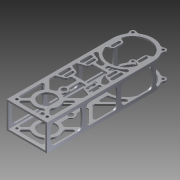
# Autodesk Inventor part: upper gearbox frame 5
Saved by Autodesk Inventor 2012 (Build 160160000, 160)
## iProperties
Created: 2013-09-11
Part Number: upper gearbox frame 5
Material: Default
Document SubType Name: Modeling
Designer: Bryce
Density: 1 g/cm^3
Author: Bryce
Autodesk Inventor part; units mm, degrees
ref_plane "YZ Plane" through (0, 0, 0) normal (1, 0, 0) x (0, 1, 0)
ref_plane "XZ Plane" through (0, 0, 0) normal (0, 1, 0) x (-1, 0, 0)
ref_plane "XY Plane" through (0, 0, 0) normal (0, 0, 1) x (1, 0, 0)
sketch "Sketch1" plane through (0, 0, 0) normal (0, 0, 1) x (1, 0, 0)
  line L0 (0, 0) -> (76.2, 0)
  line L1 (76.2, 0) -> (76.2, 50.8)
  line L2 (76.2, 50.8) -> (0, 50.8)
  line L3 (0, 50.8) -> (0, 0)
  line L4 (3.175, 3.175) -> (73.025, 3.175)
  line L5 (73.025, 3.175) -> (73.025, 47.625)
  line L6 (73.025, 47.625) -> (3.175, 47.625)
  line L7 (3.175, 47.625) -> (3.175, 3.175)
  dimension "d0" = 50.8
  dimension "d1" = 76.2
  dimension "d2" = 3.175
  dimension "d3" = 3.175
  dimension "d4" = 3.175
  dimension "d5" = 3.175
  constraints: 16 end point, 4 parallel, 2 horizontal, 2 perpendicular
  measures "d0" distance of L2.end L0.start
  measures "d1" distance of L0.start L0.end
  measures "d2" distance between parallel lines of L0 L4
  measures "d3" distance between parallel lines of L3 L7
  measures "d4" distance between parallel lines of L2 L6
  measures "d5" distance between parallel lines of L1 L5
extrude "Extrusion1" add sketch "Sketch1" along normal blind 254
sketch "Sketch2" plane through (0, 0, 0) normal (0, -1, 0) x (1, 0, 0)
  line L0 (76.2, 254) -> (0, 254) projected
  line L1 (0, 0) -> (0, 254) projected
  line L2 (0, 0) -> (76.2, 0) projected
  line L3 (76.2, 0) -> (76.2, 254) projected
  circle A0 centre (38.1, 215.9) radius 15.875
  arc A1 (71.4375, 66.675) -> (4.7625, 66.675) centre (38.1, 66.675) ccw
  arc A2 (4.7625, 53.975) -> (71.4375, 53.975) centre (38.1, 53.975) ccw
  circle A3 centre (38.1, 171.45) radius 4.6482
  line L4 (38.1, 215.9) -> (0, 254) construction
  line L5 (38.1, 215.9) -> (76.2, 254) construction
  line L6 (38.1, 215.9) -> (0, 177.8) construction
  line L7 (38.1, 215.9) -> (76.2, 177.8) construction
  arc A4 (20.3007, 229.2092) -> (20.3007, 202.5908) centre (38.1, 215.9) ccw
  arc A5 (51.4092, 233.6993) -> (24.7908, 233.6993) centre (38.1, 215.9) ccw
  arc A6 (55.8993, 202.5908) -> (55.8993, 229.2092) centre (38.1, 215.9) ccw
  arc A7 (24.7908, 198.1007) -> (34.925, 193.903) centre (38.1, 215.9) ccw
  line L8 (6.35, 243.1599) -> (6.35, 188.6401)
  line L9 (10.8401, 247.65) -> (65.3599, 247.65)
  line L10 (69.85, 243.1599) -> (69.85, 188.6401)
  line L11 (6.35, 243.1599) -> (20.3007, 229.2092)
  line L12 (20.3007, 202.5908) -> (6.35, 188.6401)
  line L13 (24.7908, 233.6993) -> (10.8401, 247.65)
  line L14 (51.4092, 233.6993) -> (65.3599, 247.65)
  line L15 (69.85, 243.1599) -> (55.8993, 229.2092)
  line L16 (55.8993, 202.5908) -> (69.85, 188.6401)
  line L17 (6.35, 179.6599) -> (6.35, 168.4676)
  line L18 (69.85, 179.6599) -> (69.85, 168.4676)
  arc A8 (69.85, 87.7356) -> (41.275, 104.6425) centre (38.1, 66.675) ccw
  line L19 (6.35, 179.6599) -> (24.7908, 198.1007)
  line L20 (51.4092, 198.1007) -> (69.85, 179.6599)
  arc A9 (34.925, 178.7248) -> (34.925, 164.1752) centre (38.1, 171.45) ccw
  arc A10 (41.275, 164.1752) -> (41.275, 178.7248) centre (38.1, 171.45) ccw
  line L21 (38.1, 215.9) -> (38.1, 171.45) construction
  line L22 (38.1, 171.45) -> (38.1, 66.675) construction
  line L23 (34.925, 178.7248) -> (34.925, 193.903)
  line L24 (41.275, 193.903) -> (41.275, 178.7248)
  line L25 (34.925, 164.1752) -> (34.925, 139.8926)
  line L26 (41.275, 164.1752) -> (41.275, 139.8926)
  arc A11 (41.275, 193.903) -> (51.4092, 198.1007) centre (38.1, 215.9) ccw
  arc A12 (34.925, 193.903) -> (41.275, 193.903) centre (38.1, 215.9) ccw
  arc A13 (41.275, 104.6425) -> (34.925, 104.6425) centre (38.1, 66.675) ccw construction
  arc A14 (34.925, 104.6425) -> (6.35, 87.7356) centre (38.1, 66.675) ccw
  line L27 (4.7625, 66.675) -> (4.7625, 53.975)
  line L28 (71.4375, 66.675) -> (71.4375, 53.975)
  arc A15 (0, 53.975) -> (5.274, 34.6342) centre (38.1, 53.975) ccw
  line L29 (76.2, 95.25) -> (38.1, 133.35) construction
  line L30 (0, 95.25) -> (38.1, 133.35) construction
  line L31 (38.1, 133.35) -> (0, 171.45) construction
  line L32 (38.1, 133.35) -> (76.2, 171.45) construction
  line L33 (41.4676, 133.35) -> (69.85, 161.7324)
  line L34 (41.4676, 133.35) -> (69.85, 104.9676)
  line L35 (69.85, 98.2324) -> (41.275, 126.8074)
  line L36 (38.1, 129.9824) -> (34.925, 126.8074) construction
  line L37 (6.35, 104.9676) -> (34.7324, 133.35)
  line L38 (34.7324, 133.35) -> (6.35, 161.7324)
  line L39 (6.35, 168.4676) -> (34.925, 139.8926)
  line L40 (38.1, 136.7176) -> (41.275, 139.8926)
  line L41 (41.275, 139.8926) -> (41.275, 126.8074) construction
  line L42 (41.275, 126.8074) -> (41.275, 104.6425)
  line L43 (34.925, 126.8074) -> (34.925, 104.6425)
  line L44 (34.925, 139.8926) -> (34.925, 126.8074) construction
  line L45 (34.925, 126.8074) -> (6.35, 98.2324)
  line L46 (41.275, 126.8074) -> (38.1, 129.9824) construction
  line L47 (41.275, 139.8926) -> (69.85, 168.4676)
  line L48 (34.925, 139.8926) -> (38.1, 136.7176)
  line L49 (69.85, 161.7324) -> (69.85, 104.9676)
  line L50 (69.85, 168.4676) -> (69.85, 161.7324) construction
  line L51 (6.35, 168.4676) -> (6.35, 161.7324) construction
  line L52 (6.35, 161.7324) -> (6.35, 104.9676)
  line L53 (6.35, 104.9676) -> (6.35, 98.2324) construction
  line L54 (6.35, 98.2324) -> (6.35, 87.7356)
  line L55 (69.85, 98.2324) -> (69.85, 87.7356)
  line L56 (69.85, 104.9676) -> (69.85, 98.2324) construction
  circle A16 centre (66.675, 244.475) radius 2.5527
  circle A17 centre (66.675, 25.4) radius 2.5527
  arc A18 (64.0036, 21.0791) -> (57.4408, 21.149) centre (60.6643, 15.6781) ccw
  arc A19 (70.926, 34.6342) -> (70.9959, 28.0714) centre (76.3969, 31.4107) ccw
  arc A20 (64.0036, 21.0791) -> (70.9959, 28.0714) centre (66.675, 25.4) ccw
  arc A21 (70.926, 34.6342) -> (76.2, 53.975) centre (38.1, 53.975) ccw
  circle A22 centre (9.525, 25.4) radius 2.5527
  arc A23 (5.2041, 28.0714) -> (12.1964, 21.0791) centre (9.525, 25.4) ccw
  arc A24 (5.2041, 28.0714) -> (5.274, 34.6342) centre (-0.1969, 31.4107) ccw
  arc A25 (18.7592, 21.149) -> (12.1964, 21.0791) centre (15.5357, 15.6781) ccw
  arc A26 (18.7592, 21.149) -> (57.4408, 21.149) centre (38.1, 53.975) ccw
  circle A27 centre (9.525, 244.475) radius 2.5527
  dimension "d62" = 12.7
  dimension "d8" = 31.75
  dimension "d9" = 38.1
  dimension "d10" = 38.1
  dimension "d11" = 33.3375
  dimension "d15" = 38.1
  dimension "d18" = 12.7
  dimension "d30" = 9.2964
  dimension "d31" = 44.45
  dimension "d32" = 3.175
  dimension "d33" = 3.175
  dimension "d34" = 3.175
  dimension "d35" = 3.175
  dimension "d36" = 3.175
  dimension "d37" = 3.175
  dimension "d38" = 6.35
  dimension "d39" = 6.35
  dimension "d41" = 6.35
  dimension "d42" = 22.225
  dimension "d43" = 38.1
  dimension "d44" = 3.175
  dimension "d45" = 3.175
  dimension "d46" = 3.175
  dimension "d47" = 3.175
  dimension "d48" = 7.9375
  dimension "d202" = 120.65
  dimension "d203" = 45
  dimension "d204" = 2.3813
  dimension "d205" = 4.7625
  dimension "d206" = 4.7625
  dimension "d211" = 9.525
  dimension "d212" = 5.1054
  dimension "d213" = 228.6
  dimension "d214" = 9.525
  dimension "d216" = 6.35
  dimension "d218" = 9.525
  dimension "d237" = 187.325
  dimension "d238" = 5.08
  constraints: 106 end point, 63 parallel, 48 point on circle, 28 centre point, 25 collinear, 21 point on line, 16 perpendicular, 14 tangent, 11 equal radius, 10 coincident, 2 horizontal alignment, 1 vertical alignment
  measures "d8" diameter of A0
  measures "d9" distance from line of L1 L4.start
  measures "d10" distance from line of L0 L4.start
  measures "d11" radius of A1
  measures "d15" distance from line of L1 A1.centre
  measures "d18" distance of A1.centre A2.centre
  measures "d30" diameter of A3
  measures "d31" distance of L4.start A3.centre
  measures "d32" distance between parallel lines of L4 L11
  measures "d33" distance between parallel lines of L12 L6
  measures "d34" distance between parallel lines of L5 L14
  measures "d35" distance between parallel lines of L15 L5
  measures "d36" distance between parallel lines of L7 L16
  measures "d37" distance between parallel lines of L4 L13
  measures "d38" distance between parallel lines of L1 L8
  measures "d39" distance between parallel lines of L0 L9
  measures "d41" distance between parallel lines of L3 L10
  measures "d42" radius of A6
  measures "d43" radius of A8
  measures "d44" distance between parallel lines of L6 L19
  measures "d45" distance between parallel lines of L7 L20
  measures "d46" distance between parallel lines of L22 L25
  measures "d47" distance between parallel lines of L26 L22
  measures "d48" radius of A10
  measures "d202" distance from line of L0 L29.end
  measures "d203" angle of L3 L29
  measures "d204" distance between parallel lines of L29 L34
  measures "d205" distance between parallel lines of L34 L35
  measures "d206" distance between parallel lines of L37 L36
  measures "d211" distance from line of L0 A16.centre
  measures "d212" diameter of A16
  measures "d213" distance from line of L0 A17.centre
  measures "d214" distance from line of L3 A17.centre
  measures "d216" radius of A19
  measures "d218" distance from line of L1 A22.centre
  measures "d237" distance from line of L0 L22.end
  measures "d238" radius of A20
extrude "Extrusion2" cut sketch "Sketch2" against normal blind 6.35 contours A0 | L28 A2 L27 A1 | A3 | A4 L12 L8 L11 | A5 L13 L9 L14 | A6 L15 L10 L16 | A7 L23 A9 L25 L39 L17 L19 | A11 L20 L18 L47 L26 A10 L24 | A8 L42 L35 L55 | A14 L54 L45 L43 | L33 L49 L34 | L52 L38 L37
fillet "Fillet1" radius 3.175 40 edges at (6.35, 1.5875, 87.7356) (69.85, 1.5875, 87.7356) (34.925, 1.5875, 104.6425) (41.275, 1.5875, 104.6425) (6.35, 1.5875, 243.1599) (6.35, 1.5875, 188.6401) (6.35, 1.5875, 179.6599) (10.8401, 1.5875, 247.65) (20.3007, 1.5875, 229.2092) (20.3007, 1.5875, 202.5908) (24.7908, 1.5875, 233.6993) (34.925, 1.5875, 193.903) (34.925, 1.5875, 178.7248) (34.925, 1.5875, 164.1752) (41.275, 1.5875, 193.903) (41.275, 1.5875, 178.7248) (41.275, 1.5875, 164.1752) (51.4092, 1.5875, 233.6993) (55.8993, 1.5875, 229.2092) (51.4092, 1.5875, 198.1007) (55.8993, 1.5875, 202.5908) (65.3599, 1.5875, 247.65) (69.85, 1.5875, 243.1599) (69.85, 1.5875, 188.6401) (69.85, 1.5875, 179.6599) (24.7908, 1.5875, 198.1007) (69.85, 1.5875, 168.4676) (6.35, 1.5875, 168.4676) (69.85, 1.5875, 161.7324) (6.35, 1.5875, 161.7324) (41.275, 1.5875, 139.8926) (34.925, 1.5875, 139.8926) (41.4676, 1.5875, 133.35) (34.7324, 1.5875, 133.35) (41.275, 1.5875, 126.8074) (34.925, 1.5875, 126.8074) (69.85, 1.5875, 104.9676) (6.35, 1.5875, 104.9676) (69.85, 1.5875, 98.2324) (6.35, 1.5875, 98.2324)
sketch "Sketch3" plane through (0, 50.8, 0) normal (0, 1, 0) x (1, 0, 0)
  line L0 (0, -254) -> (76.2, -254) projected
  line L1 (76.2, 0) -> (76.2, -254) projected
  line L2 (76.2, 0) -> (0, 0) projected
  line L3 (0, 0) -> (0, -254) projected
  circle A0 centre (38.1, -215.9) radius 15.875 projected
  arc A1 (20.32, -106.68) -> (15.24, -106.68) centre (17.78, -106.68) ccw
  arc A2 (15.24, -119.38) -> (20.32, -119.38) centre (17.78, -119.38) ccw
  line L4 (20.32, -106.68) -> (20.32, -119.38)
  line L5 (15.24, -106.68) -> (15.24, -119.38)
  arc A3 (60.96, -106.68) -> (55.88, -106.68) centre (58.42, -106.68) ccw
  arc A4 (55.88, -119.38) -> (60.96, -119.38) centre (58.42, -119.38) ccw
  line L6 (60.96, -106.68) -> (60.96, -119.38)
  line L7 (55.88, -106.68) -> (55.88, -119.38)
  arc A5 (20.32, -147.32) -> (15.24, -147.32) centre (17.78, -147.32) ccw
  arc A6 (15.24, -160.02) -> (20.32, -160.02) centre (17.78, -160.02) ccw
  line L8 (20.32, -147.32) -> (20.32, -160.02)
  line L9 (15.24, -147.32) -> (15.24, -160.02)
  arc A7 (60.96, -147.32) -> (55.88, -147.32) centre (58.42, -147.32) ccw
  line L10 (60.96, -147.32) -> (60.96, -160.02)
  line L11 (55.88, -147.32) -> (55.88, -160.02)
  arc A8 (55.88, -160.02) -> (60.96, -160.02) centre (58.42, -160.02) ccw
  arc A9 (50.8, -127) -> (25.4, -127) centre (38.1, -127) ccw construction
  line L12 (50.8, -127) -> (50.8, -139.7) construction
  line L13 (25.4, -127) -> (25.4, -139.7) construction
  arc A10 (25.4, -139.7) -> (50.8, -139.7) centre (38.1, -139.7) ccw construction
  arc A11 (15.24, -53.975) -> (10.16, -53.975) centre (12.7, -53.975) ccw
  arc A12 (66.04, -53.975) -> (60.96, -53.975) centre (63.5, -53.975) ccw
  arc A13 (60.96, -66.675) -> (66.04, -66.675) centre (63.5, -66.675) ccw
  line L14 (10.16, -53.975) -> (10.16, -66.675)
  line L15 (15.24, -53.975) -> (15.24, -66.675)
  line L16 (60.96, -53.975) -> (60.96, -66.675)
  line L17 (66.04, -53.975) -> (66.04, -66.675)
  line L18 (12.7, -165.1) -> (63.5, -165.1) construction
  line L19 (63.5, -165.1) -> (63.5, -163.8962) construction
  line L20 (63.5, -101.6) -> (12.7, -101.6) construction
  line L21 (12.7, -101.6) -> (12.7, -102.8038) construction
  arc A14 (6.35, -87.7356) -> (69.85, -87.7356) centre (38.1, -66.675) ccw construction
  line L22 (6.35, -6.35) -> (69.85, -6.35) construction
  line L23 (69.85, -6.35) -> (69.85, -84.7055) construction
  line L24 (69.85, -247.65) -> (65.3599, -247.65) construction
  line L25 (6.35, -247.65) -> (6.35, -243.1599) construction
  arc A15 (10.16, -66.675) -> (15.24, -66.675) centre (12.7, -66.675) ccw
  arc A16 (76.2, -53.975) -> (0, -53.975) centre (38.1, -53.975) ccw
  circle A17 centre (38.1, -215.9) radius 31.75 construction
  circle A18 centre (38.1, -184.15) radius 4.6482
  arc A19 (24.7908, -233.6993) -> (51.4092, -233.6993) centre (38.1, -215.9) ccw
  line L26 (38.1, -215.9) -> (0, -254) construction
  line L27 (38.1, -215.9) -> (0, -177.8) construction
  line L28 (38.1, -215.9) -> (76.2, -254) construction
  line L29 (38.1, -215.9) -> (76.2, -177.8) construction
  line L30 (24.7908, -233.6993) -> (10.8401, -247.65)
  line L31 (51.4092, -233.6993) -> (65.3599, -247.65)
  line L32 (65.3599, -247.65) -> (10.8401, -247.65)
  line L33 (10.8401, -247.65) -> (6.35, -247.65) construction
  line L34 (20.3007, -229.2092) -> (6.35, -243.1599)
  line L35 (20.3007, -202.5908) -> (6.35, -188.6401)
  line L36 (24.7908, -198.1007) -> (6.35, -179.6599)
  line L37 (51.4092, -198.1007) -> (69.85, -179.6599)
  line L38 (55.8993, -202.5908) -> (69.85, -188.6401)
  line L39 (55.8993, -229.2092) -> (69.85, -243.1599)
  arc A20 (20.3007, -202.5908) -> (20.3007, -229.2092) centre (38.1, -215.9) ccw
  arc A21 (51.4092, -198.1007) -> (44.851, -194.7251) centre (38.1, -215.9) ccw
  arc A22 (55.8993, -229.2092) -> (55.8993, -202.5908) centre (38.1, -215.9) ccw
  line L40 (69.85, -188.6401) -> (69.85, -243.1599)
  line L41 (69.85, -243.1599) -> (69.85, -247.65) construction
  line L42 (6.35, -243.1599) -> (6.35, -188.6401)
  line L43 (6.35, -188.6401) -> (6.35, -179.6599) construction
  arc A23 (19.5175, -164.7936) -> (22.86, -160.02) centre (17.78, -160.02) ccw
  arc A24 (22.86, -147.32) -> (19.5175, -142.5464) centre (17.78, -147.32) ccw
  arc A25 (19.5175, -124.1536) -> (22.86, -119.38) centre (17.78, -119.38) ccw
  arc A26 (22.86, -106.68) -> (19.5175, -101.9064) centre (17.78, -106.68) ccw
  arc A27 (56.6825, -101.9064) -> (53.34, -106.68) centre (58.42, -106.68) ccw
  arc A28 (53.34, -119.38) -> (56.6825, -124.1536) centre (58.42, -119.38) ccw
  arc A29 (56.6825, -142.5464) -> (53.34, -147.32) centre (58.42, -147.32) ccw
  arc A30 (53.34, -160.02) -> (56.6825, -164.7936) centre (58.42, -160.02) ccw
  line L44 (22.86, -147.32) -> (22.86, -151.2887)
  line L45 (22.86, -106.68) -> (22.86, -110.6487)
  line L46 (53.34, -106.68) -> (53.34, -110.6487)
  line L47 (53.34, -147.32) -> (53.34, -151.2887)
  line L48 (19.5175, -142.5464) -> (6.35, -137.7538)
  line L49 (19.5175, -124.1536) -> (6.35, -128.9462)
  line L50 (56.6825, -124.1536) -> (69.85, -128.9462)
  line L51 (56.6825, -142.5464) -> (69.85, -137.7538)
  line L52 (19.5175, -101.9064) -> (6.35, -97.1138)
  line L53 (56.6825, -101.9064) -> (69.85, -97.1138)
  line L54 (19.5175, -164.7936) -> (6.35, -169.5862)
  line L55 (56.6825, -164.7936) -> (69.85, -169.5862)
  line L56 (22.86, -153.67) -> (53.34, -153.67) construction
  line L57 (22.86, -113.03) -> (53.34, -113.03) construction
  line L58 (22.86, -115.4112) -> (53.34, -115.4112)
  line L59 (22.86, -110.6487) -> (35.7188, -110.6487)
  line L60 (22.86, -151.2887) -> (53.34, -151.2887)
  line L61 (22.86, -156.0512) -> (35.7188, -156.0512)
  arc A31 (35.7188, -176.9116) -> (32.6538, -189.4795) centre (38.1, -184.15) ccw
  arc A32 (43.5462, -189.4795) -> (40.4813, -176.9116) centre (38.1, -184.15) ccw
  line L62 (38.1, -153.67) -> (38.1, -184.15) construction
  line L63 (35.7188, -156.0512) -> (35.7188, -176.9116)
  line L64 (40.4813, -156.0512) -> (40.4813, -176.9116)
  arc A33 (31.349, -194.7251) -> (32.6538, -189.4795) centre (30.3846, -191.7002) ccw
  arc A34 (31.349, -194.7251) -> (24.7908, -198.1007) centre (38.1, -215.9) ccw
  arc A35 (44.851, -194.7251) -> (31.349, -194.7251) centre (38.1, -215.9) ccw construction
  line L65 (35.7188, -156.0512) -> (40.4813, -156.0512) construction
  line L66 (40.4813, -156.0512) -> (53.34, -156.0512)
  line L67 (6.35, -169.5862) -> (6.35, -141.1326)
  line L68 (6.35, -179.6599) -> (6.35, -169.5862)
  line L69 (69.85, -179.6599) -> (69.85, -188.6401) construction
  line L70 (69.85, -169.5862) -> (69.85, -179.6599)
  line L71 (69.85, -137.7538) -> (69.85, -141.1326) construction
  line L72 (6.35, -137.7538) -> (6.35, -128.9462)
  line L73 (69.85, -128.9462) -> (69.85, -137.7538)
  arc A36 (69.85, -53.975) -> (68.9758, -46.5759) centre (38.1, -53.975) ccw construction
  arc A37 (14.4375, -71.4486) -> (17.78, -66.675) centre (12.7, -66.675) ccw
  arc A38 (17.78, -53.975) -> (14.4375, -49.2014) centre (12.7, -53.975) ccw
  arc A39 (61.7625, -49.2014) -> (58.42, -53.975) centre (63.5, -53.975) ccw
  arc A40 (58.42, -66.675) -> (61.7625, -71.4486) centre (63.5, -66.675) ccw
  line L74 (17.78, -53.975) -> (17.78, -66.675)
  line L75 (58.42, -53.975) -> (58.42, -66.675)
  line L76 (14.4375, -71.4486) -> (7.2242, -74.0741)
  line L77 (14.4375, -49.2014) -> (7.2242, -46.5759)
  line L78 (61.7625, -49.2014) -> (68.9758, -46.5759)
  line L79 (61.7625, -71.4486) -> (68.9758, -74.0741)
  arc A41 (6.35, -66.675) -> (7.2242, -74.0741) centre (38.1, -66.675) ccw construction
  arc A42 (7.2242, -74.0741) -> (68.9758, -74.0741) centre (38.1, -66.675) ccw
  line L80 (7.2242, -74.0741) -> (10.16, -73.0055)
  arc A43 (68.9758, -74.0741) -> (69.85, -66.675) centre (38.1, -66.675) ccw construction
  arc A44 (7.2242, -46.5759) -> (6.35, -53.975) centre (38.1, -53.975) ccw construction
  arc A45 (68.9758, -46.5759) -> (7.2242, -46.5759) centre (38.1, -53.975) ccw
  arc A46 (6.35, -84.7055) -> (35.7188, -103.1098) centre (38.1, -66.675) ccw
  line L81 (38.1, -103.1875) -> (38.1, -110.6487) construction
  line L82 (35.7188, -103.1098) -> (35.7188, -110.6487)
  line L83 (40.4813, -110.6487) -> (40.4813, -103.1098)
  arc A47 (35.7188, -103.1098) -> (40.4813, -103.1098) centre (38.1, -66.675) ccw construction
  arc A48 (40.4813, -103.1098) -> (69.85, -84.7055) centre (38.1, -66.675) ccw
  line L84 (35.7188, -110.6487) -> (40.4813, -110.6487) construction
  line L85 (40.4813, -110.6487) -> (53.34, -110.6487)
  line L86 (22.86, -115.4112) -> (22.86, -119.38)
  line L87 (22.86, -110.6487) -> (22.86, -115.4112) construction
  line L88 (53.34, -110.6487) -> (53.34, -115.4112) construction
  line L89 (53.34, -115.4112) -> (53.34, -119.38)
  line L90 (22.86, -151.2887) -> (22.86, -156.0512) construction
  line L91 (22.86, -156.0512) -> (22.86, -160.02)
  line L92 (53.34, -156.0512) -> (53.34, -160.02)
  line L93 (53.34, -151.2887) -> (53.34, -156.0512) construction
  line L94 (6.35, -97.1138) -> (6.35, -84.7055)
  line L95 (6.35, -84.7055) -> (6.35, -6.35) construction
  line L96 (69.85, -84.7055) -> (69.85, -97.1138)
  line L97 (69.85, -97.1138) -> (69.85, -100.4926) construction
  line L98 (12.7, -163.8962) -> (6.35, -166.2074)
  line L99 (12.7, -143.4438) -> (6.35, -141.1326)
  line L100 (12.7, -123.2562) -> (6.35, -125.5674)
  line L101 (12.7, -102.8038) -> (6.35, -100.4926)
  line L102 (63.5, -102.8038) -> (69.85, -100.4926)
  line L103 (63.5, -123.2562) -> (69.85, -125.5674)
  line L104 (63.5, -163.8962) -> (69.85, -166.2074)
  line L105 (63.5, -143.4438) -> (69.85, -141.1326)
  line L106 (12.7, -163.8962) -> (12.7, -165.1) construction
  line L107 (12.7, -143.4438) -> (12.7, -163.8962)
  line L108 (63.5, -163.8962) -> (63.5, -143.4438)
  line L109 (63.5, -143.4438) -> (63.5, -123.2562) construction
  line L110 (12.7, -102.8038) -> (12.7, -123.2562)
  line L111 (12.7, -123.2562) -> (12.7, -143.4438) construction
  line L112 (63.5, -102.8038) -> (63.5, -101.6) construction
  line L113 (63.5, -123.2562) -> (63.5, -102.8038)
  line L114 (69.85, -100.4926) -> (69.85, -125.5674)
  line L115 (69.85, -125.5674) -> (69.85, -128.9462) construction
  line L116 (6.35, -100.4926) -> (6.35, -125.5674)
  line L117 (6.35, -100.4926) -> (6.35, -97.1138) construction
  line L118 (6.35, -125.5674) -> (6.35, -128.9462) construction
  line L119 (69.85, -141.1326) -> (69.85, -166.2074)
  line L120 (69.85, -166.2074) -> (69.85, -169.5862) construction
  line L121 (6.35, -141.1326) -> (6.35, -137.7538) construction
  circle A49 centre (38.1, -184.15) radius 15.875 construction
  arc A50 (43.5462, -189.4795) -> (44.851, -194.7251) centre (45.8154, -191.7002) ccw
  dimension "d91" = 63.5
  dimension "d52" = 12.7
  dimension "d53" = 2.54
  dimension "d54" = 12.7
  dimension "d55" = 2.54
  dimension "d56" = 12.7
  dimension "d57" = 2.54
  dimension "d58" = 12.7
  dimension "d59" = 2.54
  dimension "d60" = 40.64
  dimension "d61" = 40.64
  dimension "d62" = 12.7
  dimension "d63" = 12.7
  dimension "d64" = 20.32
  dimension "d65" = 20.32
  dimension "d66" = 76.2
  dimension "d70" = 2.54
  dimension "d71" = 50.8
  dimension "d74" = 50.8
  dimension "d75" = 63.5
  dimension "d76" = 5.08
  dimension "d77" = 5.08
  dimension "d78" = 38.1
  dimension "d79" = 6.35
  dimension "d80" = 6.35
  dimension "d81" = 6.35
  dimension "d82" = 6.35
  dimension "d83" = 2.54
  dimension "d86" = 12.7
  dimension "d87" = 12.7
  dimension "d89" = 25.4
  dimension "d90" = 187.325
  dimension "d92" = 9.2964
  dimension "d94" = 3.175
  dimension "d95" = 3.175
  dimension "d96" = 22.225
  dimension "d97" = 6.35
  dimension "d98" = 6.35
  dimension "d99" = 6.35
  dimension "d100" = 3.175
  dimension "d101" = 3.175
  dimension "d102" = 6.35
  dimension "d103" = 5.08
  dimension "d106" = 4.7625
  dimension "d107" = 2.3813
  dimension "d108" = 4.7625
  dimension "d109" = 2.3813
  dimension "d110" = 2.3813
  dimension "d111" = 4.7625
  dimension "d112" = 7.62
  dimension "d113" = 3.175
  dimension "d115" = 70
  dimension "d116" = 5.08
  dimension "d119" = 36.5125
  dimension "d120" = 4.7625
  dimension "d121" = 2.3813
  dimension "d123" = 30.48
  dimension "d124" = 70
  dimension "d125" = 70
  dimension "d192" = 3.175
  dimension "d193" = 3.175
  dimension "d194" = 3.175
  dimension "d195" = 3.175
  dimension "d196" = 3.175
  dimension "d197" = 3.175
  constraints: 236 end point, 207 parallel, 101 point on circle, 77 tangent, 49 centre point, 44 point on line, 38 perpendicular, 24 coincident, 23 collinear, 16 equal radius, 8 vertical alignment, 5 horizontal alignment, 5 midpoint, 4 horizontal, 2 vertical, 2 other
  measures "d52" distance of A2.centre A1.centre
  measures "d53" radius of A1
  measures "d54" distance of A4.centre A3.centre
  measures "d55" radius of A3
  measures "d56" distance of A6.centre A5.centre
  measures "d57" radius of A5
  measures "d58" distance of A8.centre A7.centre
  measures "d59" radius of A7
  measures "d60" distance of A3.centre A1.centre
  measures "d61" distance of A2.centre A6.centre
  measures "d62" distance of A10.centre A9.centre
  measures "d63" radius of A9
  measures "d64" horizontal distance of A1.centre A9.centre
  measures "d65" horizontal distance of A1.centre A9.centre
  measures "d66" distance of A0.centre A10.centre
  measures "d70" radius of A12
  measures "d71" distance of A12.centre A11.centre
  measures "d74" distance of L20.start L20.end
  measures "d75" distance of L20.end L18.start
  measures "d76" distance from line of L20 A1.centre
  measures "d77" distance from line of L21 A1.centre
  measures "d78" radius of A14
  measures "d79" distance between parallel lines of L3 L25
  measures "d80" distance between parallel lines of L0 L24
  measures "d81" distance between parallel lines of L1 L23
  measures "d82" distance between parallel lines of L2 L22
  measures "d83" radius of A11
  measures "d86" distance of A14.centre A16.centre
  measures "d87" distance of L14.start L14.end
  measures "d89" distance of A11.centre A16.centre
  measures "d90" distance from line of L0 A14.centre
  measures "d92" diameter of A18
  measures "d94" distance between parallel lines of L30 L26
  measures "d95" distance between parallel lines of L28 L31
  measures "d96" radius of A19
  measures "d97" distance between parallel lines of L30 L34
  measures "d98" distance between parallel lines of L36 L35
  measures "d99" distance between parallel lines of L38 L37
  measures "d100" distance between parallel lines of L29 L37
  measures "d101" distance between parallel lines of L27 L36
  measures "d102" distance between parallel lines of L39 L31
  measures "d103" radius of A29
  measures "d106" distance of L45.end L58.start
  measures "d107" distance of L57.end L58.end
  measures "d108" distance of L61.start L44.end
  measures "d109" distance of L56.end L66.end
  measures "d110" distance between parallel lines of L64 L62
  measures "d111" distance between parallel lines of L64 L63
  measures "d112" radius of A31
  measures "d113" radius of A33
  measures "d115" angle of L67 L48
  measures "d116" radius of A37
  measures "d119" radius of A46
  measures "d120" distance between parallel lines of L83 L82
  measures "d121" distance of L81.end L59.end
  measures "d123" distance of L62.start L62.end
  measures "d124" angle of L76 L95
  measures "d125" angle of L95 L77
  measures "d192" distance from line of L48 L67.end
  measures "d193" distance between parallel lines of L54 L98
  measures "d194" distance from line of L49 L100.end
  measures "d195" distance from line of L52 L101.end
  measures "d196" distance between parallel lines of L53 L102
  measures "d197" distance from line of L50 L103.end
extrude "Extrusion3" cut sketch "Sketch2" against normal through all contours L3 L2 L1 A15 A24 A23 A25 A26 A18 A20 A19 A21
extrude "Extrusion4" cut sketch "Sketch3" against normal blind 3.175 contours A0 | L4 A2 L5 A1 | L6 A4 L7 A3 | L8 A6 L9 A5 | L10 A8 L11 A7 | L15 A15 L14 A11 | L17 A13 L16 A12 | A18 | A19 L31 L32 L30 | L34 L42 L35 A20 | L36 L68 L54 A23 L91 L61 L63 A31 A33 A34 | A21 A50 A32 L64 L66 L92 A30 L55 L70 L37 | L38 L40 L39 A22 | A24 L48 L72 L49 A25 L86 L58 L89 A28 L50 L73 L51 A29 L47 L60 L44 | A26 L52 L94 A46 L82 L59 L45 | A27 L46 L85 L83 A48 L96 L53 | L67 L99 L107 L98 | A37 L74 A38 L77 A45 L78 A39 L75 A40 L79 A42 L76 | L100 L116 L101 L110 | L102 L114 L103 L113 | L108 L105 L119 L104
fillet "Fillet2" radius 3.175 62 edges at (65.3599, 49.2125, 247.65) (10.8401, 49.2125, 247.65) (51.4092, 49.2125, 233.6993) (24.7908, 49.2125, 233.6993) (55.8993, 49.2125, 229.2092) (20.3007, 49.2125, 229.2092) (69.85, 49.2125, 243.1599) (6.35, 49.2125, 243.1599) (55.8993, 49.2125, 202.5908) (20.3007, 49.2125, 202.5908) (51.4092, 49.2125, 198.1007) (24.7908, 49.2125, 198.1007) (69.85, 49.2125, 188.6401) (6.35, 49.2125, 188.6401) (69.85, 49.2125, 179.6599) (6.35, 49.2125, 179.6599) (40.4813, 49.2125, 176.9116) (35.7188, 49.2125, 176.9116) (69.85, 49.2125, 169.5862) (6.35, 49.2125, 169.5862) (53.34, 49.2125, 156.0512) (40.4812, 49.2125, 156.0512) (35.7187, 49.2125, 156.0512) (22.86, 49.2125, 156.0512) (53.34, 49.2125, 151.2887) (22.86, 49.2125, 151.2887) (69.85, 49.2125, 137.7538) (6.35, 49.2125, 137.7538) (69.85, 49.2125, 128.9462) (6.35, 49.2125, 128.9462) (53.34, 49.2125, 115.4112) (22.86, 49.2125, 115.4112) (53.34, 49.2125, 110.6487) (40.4813, 49.2125, 110.6487) (35.7188, 49.2125, 110.6487) (22.86, 49.2125, 110.6487) (40.4812, 49.2125, 103.1098) (35.7188, 49.2125, 103.1098) (69.85, 49.2125, 84.7055) (6.35, 49.2125, 84.7055) (68.9758, 49.2125, 74.0741) (7.2242, 49.2125, 74.0741) (68.9758, 49.2125, 46.5759) (7.2242, 49.2125, 46.5759) (63.5, 49.2125, 163.8962) (69.85, 49.2125, 166.2074) (69.85, 49.2125, 141.1326) (63.5, 49.2125, 143.4438) (6.35, 49.2125, 141.1326) (12.7, 49.2125, 143.4438) (12.7, 49.2125, 163.8962) (6.35, 49.2125, 166.2074) (6.35, 49.2125, 125.5674) (12.7, 49.2125, 123.2562) (12.7, 49.2125, 102.8038) (6.35, 49.2125, 100.4926) (63.5, 49.2125, 123.2562) (69.85, 49.2125, 125.5674) (69.85, 49.2125, 100.4926) (63.5, 49.2125, 102.8038) (6.35, 49.2125, 97.1138) (69.85, 49.2125, 97.1138)
sketch "Sketch4" plane through (76.2, 0, 254) normal (1, 0, 0) x (0, 0, -1)
  line L0 (215.9, 50.8) -> (215.9, 0)
  line L1 (215.9, 47.625) -> (212.725, 47.625)
  line L2 (215.9, 3.175) -> (212.725, 3.175)
  line L3 (206.375, 41.275) -> (206.375, 9.525)
  arc A0 (212.725, 47.625) -> (206.375, 41.275) centre (212.725, 41.275) ccw
  arc A1 (206.375, 9.525) -> (212.725, 3.175) centre (212.725, 9.525) ccw
  line L4 (0, 50.8) -> (0, 0) projected
  line L5 (6.35, 6.35) -> (8.7697, 6.35) construction
  line L6 (200.025, 6.35) -> (200.025, 44.45)
  line L7 (200.025, 44.45) -> (64.2553, 44.45) construction
  line L8 (6.35, 44.45) -> (6.35, 25.4) construction
  arc A2 (8.7697, 44.45) -> (8.7697, 6.35) centre (82.55, 25.4) ccw
  line L9 (66.675, 44.45) -> (66.675, 6.35) construction
  arc A3 (64.2553, 6.35) -> (64.2553, 44.45) centre (-9.525, 25.4) ccw
  line L10 (69.85, 44.45) -> (69.85, 6.35) construction
  line L11 (8.7697, 6.35) -> (64.2553, 6.35)
  line L12 (6.35, 25.4) -> (6.35, 6.35) construction
  line L13 (8.7697, 44.45) -> (6.35, 44.45) construction
  line L14 (64.2553, 44.45) -> (8.7697, 44.45)
  line L15 (64.2553, 6.35) -> (200.025, 6.35) construction
  line L16 (3.175, 44.45) -> (3.175, 6.35) construction
  arc A4 (75.4447, 44.45) -> (75.4447, 6.35) centre (149.225, 25.4) ccw
  arc A5 (130.9303, 6.35) -> (130.9303, 44.45) centre (57.15, 25.4) ccw
  line L17 (75.4447, 6.35) -> (130.9303, 6.35)
  line L18 (130.9303, 44.45) -> (75.4447, 44.45)
  arc A6 (142.1197, 44.45) -> (142.1197, 6.35) centre (215.9, 25.4) ccw
  arc A7 (197.6053, 6.35) -> (197.6053, 44.45) centre (123.825, 25.4) ccw
  line L19 (142.1197, 6.35) -> (197.6053, 6.35)
  line L20 (197.6053, 44.45) -> (142.1197, 44.45)
  line L21 (200.025, 0) -> (0, 0) projected
  line L22 (200.025, 50.8) -> (0, 50.8) projected
  line L23 (200.025, 0) -> (219.3658, 0) projected
  line L24 (219.3658, 50.8) -> (200.025, 50.8) projected
  line L25 (200.025, 50.8) -> (200.025, 0) projected
  point P0 (133.35, 6.35)
  point P1 (136.525, 6.35)
  point P2 (73.025, 25.4)
  point P3 (203.2, 6.35)
  point P4 (139.7, 25.4)
  dimension "d129" = 6.35
  dimension "d133" = 3.175
  dimension "d175" = 6.35
  dimension "d179" = 76.2
  dimension "d181" = 3.175
  dimension "d183" = 3.175
  dimension "d184" = 66.675
  dimension "d187" = 66.675
  dimension "d221" = 6.35
  dimension "d222" = 15.875
  dimension "d223" = 3.175
  dimension "d224" = 3.175
  dimension "d226" = 6.35
  constraints: 40 end point, 19 point on circle, 15 point on line, 12 parallel, 9 perpendicular, 8 centre point, 8 tangent, 4 horizontal, 2 equal radius, 2 vertical alignment, 1 collinear, 26 other
  measures "d129" radius of A0
  measures "d133" distance of L1.start L1.end
  measures "d175" distance between parallel lines of L8 L4
  measures "d179" radius of A2
  measures "d181" distance between parallel lines of L10 L9
  measures "d183" distance between parallel lines of L12 L16
  measures "d184" distance between parallel lines of L10 L16
  measures "d187" distance of A2.centre A4.centre
  measures "d221" distance between parallel lines of L21 L11
  measures "d222" distance between parallel lines of L25 L0
  measures "d223" distance between parallel lines of L23 L2
  measures "d224" distance between parallel lines of L1 L24
  measures "d226" distance between parallel lines of L22 L14
extrude "Extrusion5" cut sketch "Sketch4" against normal through all contours L0 L2 A1 L3 A0 L1 | A7 L19 A6 L20 | L14 A3 L11 A2 | L18 A5 L17 A4
fillet "Fillet3" radius 6.35 24 edges at (74.6125, 44.45, 245.2303) (74.6125, 44.45, 189.7447) (74.6125, 44.45, 178.5553) (74.6125, 44.45, 123.0697) (74.6125, 44.45, 111.8803) (74.6125, 44.45, 56.3947) (74.6125, 6.35, 245.2303) (74.6125, 6.35, 189.7447) (74.6125, 6.35, 178.5553) (74.6125, 6.35, 123.0697) (74.6125, 6.35, 111.8803) (74.6125, 6.35, 56.3947) (1.5875, 6.35, 245.2303) (1.5875, 6.35, 189.7447) (1.5875, 6.35, 178.5553) (1.5875, 6.35, 123.0697) (1.5875, 6.35, 111.8803) (1.5875, 6.35, 56.3947) (1.5875, 44.45, 245.2303) (1.5875, 44.45, 189.7447) (1.5875, 44.45, 178.5553) (1.5875, 44.45, 123.0697) (1.5875, 44.45, 111.8803) (1.5875, 44.45, 56.3947)
sketch "Sketch5" plane through (0, 0, 254) normal (0, -1, 0) x (1, 0, 0)
  circle A0 centre (38.1, -82.55) radius 4.6482 projected
  arc A1 (26.8124, -57.2453) -> (32.5438, -59.6193) centre (38.1, -38.1) ccw projected
  arc A2 (34.925, -62.6934) -> (32.5438, -59.6193) centre (31.75, -62.6934) ccw projected
  line L0 (34.925, -62.6934) -> (34.925, -73.4305) projected
  arc A3 (33.5643, -76.0361) -> (34.925, -73.4305) centre (31.75, -73.4305) ccw projected
  arc A4 (33.5643, -76.0361) -> (33.5643, -89.0639) centre (38.1, -82.55) ccw projected
  arc A5 (34.925, -91.6695) -> (33.5643, -89.0639) centre (31.75, -91.6695) ccw projected
  line L1 (34.925, -91.6695) -> (34.925, -106.4423) projected
  arc A6 (29.5049, -108.6873) -> (34.925, -106.4423) centre (31.75, -106.4423) ccw projected
  line L2 (41.275, -73.4305) -> (41.275, -62.6934) projected
  arc A7 (43.6563, -59.6193) -> (41.275, -62.6934) centre (44.45, -62.6934) ccw projected
  arc A8 (41.275, -106.4423) -> (46.6951, -108.6873) centre (44.45, -106.4423) ccw projected
  line L3 (41.275, -106.4423) -> (41.275, -91.6695) projected
  arc A9 (42.6357, -89.0639) -> (41.275, -91.6695) centre (44.45, -91.6695) ccw projected
  arc A10 (42.6357, -89.0639) -> (42.6357, -76.0361) centre (38.1, -82.55) ccw projected
  arc A11 (41.275, -73.4305) -> (42.6357, -76.0361) centre (44.45, -73.4305) ccw projected
  line L4 (7.2799, -154.8377) -> (29.5049, -132.6127) projected
  arc A12 (32.5438, -59.6193) -> (43.6563, -59.6193) centre (38.1, -38.1) ccw
  line L5 (29.5049, -108.6873) -> (35.8549, -115.0373)
  line L6 (38.1, -117.2824) -> (40.3451, -115.0373) construction
  arc A13 (35.8549, -115.0373) -> (40.3451, -115.0373) centre (38.1, -112.7923) ccw
  line L7 (35.8549, -115.0373) -> (38.1, -117.2824) construction
  line L8 (40.3451, -115.0373) -> (46.6951, -108.6873)
  point P0 (0, -254)
  constraints: 8 end point, 8 tangent, 6 perpendicular, 4 point on circle, 2 centre point, 1 coincident, 1 equal radius
extrude "Extrusion6" cut sketch "Sketch5" against normal blind 1.5875
extrude "Extrusion7" cut sketch "Sketch2" against normal through all contours A16 | A17 | A22 | A27
thread "Thread1" size "1/4-20 UNC" class "2B" standard "ANSI Unified Screw Threads" full length
thread "Thread2" size "1/4-20 UNC" class "2B" standard "ANSI Unified Screw Threads" full length
thread "Thread3" size "1/4-20 UNC" class "2B" standard "ANSI Unified Screw Threads" full length
thread "Thread4" size "1/4-20 UNC" class "2B" standard "ANSI Unified Screw Threads" full length
equation "\"d2\" = d4"
equation "\"d4\" = d3"
equation "\"d5\" = d2"
equation "\"d10\" = d9"
equation "\"d32\" = d33"
equation "\"d33\" = d35"
equation "\"d34\" = d32"
equation "\"d36\" = d33"
equation "\"d37\" = d34"
equation "\"d39\" = d41"
equation "\"d41\" = d38"
equation "\"d44\" = d33"
equation "\"d45\" = d44"
equation "\"d47\" = d46"
equation "\"d61\" = d60"
equation "\"d64\" = 0.5 * d60"
equation "\"d65\" = d64"
equation "\"d77\" = d76"
equation "\"d79\" = d80"
equation "\"d80\" = d81"
equation "\"d82\" = d79"
equation "\"d83\" = d70"
body "Solid1"
